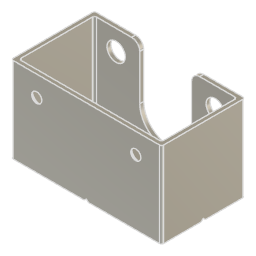
Nutdriver Holder (Autodesk Fusion 360 design; units mm, degrees)
Autodesk Fusion 360 part; units mm, degrees
sketch "Sketch1" plane through (0, 0, 0) normal (0, 0, 1) x (1, 0, 0)
  line L0 (0, 0) -> (-70, 0)
  line L1 (-70, 0) -> (-70, -37)
  line L2 (-70, -37) -> (0, -37)
  line L3 (0, -37) -> (0, 0)
  line L4 (2, 2) -> (-72, 2)
  line L5 (-72, 2) -> (-72, -39)
  line L6 (-72, -39) -> (2, -39)
  line L7 (2, -39) -> (2, 2)
  dimension "d1" = 37
  dimension "d2" = 70
  dimension "d3" = 2
  constraint horizontal L0
  constraint vertical L1
  constraint horizontal L2
  constraint vertical L3
  constraint coincident L0.start L3.end
  measures "d1" distance of L0.start L2.end
  measures "d2" distance of L0.start L0.end
extrude "Extrude1" add sketch "Sketch1" along normal blind 42
extrude "Extrude2" add sketch "Sketch1" along normal blind 2 contours L0 L1 L2 L3
fillet "Fillet1" radius 1 4 edges at (0, -37, 22) (-70, -37, 22) (-70, 0, 22) (0, 0, 22)
fillet "Fillet2" radius 1 4 edges at (2, -39, 21) (-72, -39, 21) (-72, 2, 21) (2, 2, 21)
chamfer "Chamfer1" distance 1 angle 45 8 edges at (-70, -18.5, 2) (-69.7071, -0.2929, 2) (-35, 0, 2) (-0.2929, -0.2929, 2) (0, -18.5, 2) (-0.2929, -36.7071, 2) (-35, -37, 2) (-69.7071, -36.7071, 2)
sketch "Sketch2" plane through (0, 2, 0) normal (0, 1, 0) x (-1, 0, 0)
  line L0 (-1, 42) -> (-1, 0)
  line L1 (-1, 0) -> (71, 0)
  line L2 (71, 0) -> (71, 42)
  line L3 (71, 42) -> (-1, 42)
  line L4 (35, 42) -> (35, 0) construction
  line L5 (22.2945, 42) -> (22.2945, 15.7055)
  line L6 (47.7055, 42) -> (47.7055, 15.7055)
  arc A0 (22.2945, 15.7055) -> (47.7055, 15.7055) centre (35, 15.7055) ccw
  circle A1 centre (10.6473, 32) radius 4.5
  circle A2 centre (59.3527, 32) radius 4.5
  line L7 (-1, 32) -> (22.2945, 32) construction
  dimension "d13" = 3
  dimension "d14" = 9
  dimension "d15" = 10
  constraint midpoint L3 L4.start
  constraint midpoint L1 L4.end
  constraint coincident L3 L5.start
  constraint perpendicular L3 L5
  constraint symmetric L4 L5.start L6.start
  constraint symmetric L4 L5.end L6.end
  constraint tangent L5 A0
  constraint symmetric L4 A1 A2
  constraint coincident L0 L7.start
  constraint coincident L5 L7.end
  constraint perpendicular L5 L7
  constraint midpoint A1.centre L7
  measures "d13" distance of L1 A0
  measures "d14" diameter of A1
  measures "d15" distance of L3 A1.centre
extrude "Extrude3" cut sketch "Sketch2" against normal up to surface (2 mm away) contours L3 L5 L6 A0 | A1 | A2
fillet "Fillet3" radius 4 2 edges at (-22.2945, 1, 42) (-47.7055, 1, 42)
sketch "projecting holes for attachment" plane through (0, -37, 0) normal (0, 1, 0) x (-1, 0, 0)
  line L0 (1, 3) -> (69, 3)
  line L1 (69, 3) -> (69, 42)
  line L2 (69, 42) -> (1, 42)
  line L3 (1, 42) -> (1, 3)
  point P0 (10.6473, 32)
  point P1 (59.3527, 32)
hole "Hole1" at (-59.3527, -37, 32) at (-10.6473, -37, 32) direction (0, -1, 0) diameter 5 depth 11 tip angle 118 countersink diameter 8.5 countersink angle 90
sketch "Splitting the base for printability" plane through (2, 0, 0) normal (1, 0, 0) x (0, 1, 0)
  line L0 (1, 0) -> (1, 42)
  line L1 (1, 42) -> (-38, 42)
  line L2 (-38, 42) -> (-38, 0)
  line L3 (-38, 0) -> (1, 0)
  line L4 (-38, 0) -> (1, 0)
  line L5 (-18.5, 0) -> (-18.5, 1) construction
  line L6 (-18.5, 1) -> (-19.5, 0)
  line L7 (-18.5, 1) -> (-17.5, 0)
  dimension "d26" = 1
  dimension "d27" = 90
  constraint midpoint L4 L5.start
  constraint perpendicular L4 L5
  constraint coincident L4 L6.end
  constraint symmetric L6.start L5 L7.start
  constraint symmetric L5 L6.end L7.end
  measures "d26" distance of L5.start L5.end
  measures "d27" angle of L6 L7
extrude "Extrude4" cut sketch "Splitting the base for printability" against normal up to surface (74 mm away) contours L3 L4 L6 L7
sketch "Splitting the base for printability 2" plane through (0, -39, 0) normal (0, -1, 0) x (1, 0, 0)
  circle A0 centre (-59.3527, 32) radius 2.5
  circle A1 centre (-10.6473, 32) radius 2.5
  line L0 (-71, 42) -> (-71, 0)
  line L1 (-71, 0) -> (1, 0)
  line L2 (1, 0) -> (1, 42)
  line L3 (1, 42) -> (-71, 42)
  line L4 (-35, 0) -> (-35, 1) construction
  line L5 (-35, 1) -> (-34, 0)
  line L6 (-35, 1) -> (-36, 0)
  dimension "d30" = 1
  dimension "d31" = 90
  constraint midpoint L1 L4.start
  constraint perpendicular L1 L4
  constraint coincident L1 L5.end
  constraint symmetric L5.start L4 L6.start
  constraint symmetric L4 L5.end L6.end
  measures "d30" distance of L4.start L4.end
  measures "d31" angle of L5 L6
extrude "Extrude5" cut sketch "Splitting the base for printability 2" against normal blind 41 contours L1 L5 L6
named bodies: "Nutdriver Holder"
